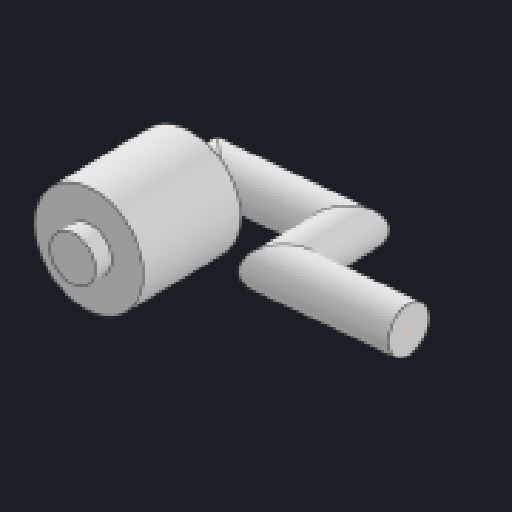
# Autodesk Inventor part: shoulder
Saved by Autodesk Inventor 2023 (Build 270158000, 158)
## iProperties
Created: 2024-02-21
Part Number: shoulder
Material: Generic
Document SubType Name: Modeling
Designer: valer
Density: 1 g/cm^3
Appearance: Default
Author: valer
Autodesk Inventor part; units mm, degrees
ref_plane "YZ Plane" through (0, 0, 0) normal (1, 0, 0) x (0, 1, 0)
ref_plane "XZ Plane" through (0, 0, 0) normal (0, 1, 0) x (-1, 0, 0)
ref_plane "XY Plane" through (0, 0, 0) normal (0, 0, 1) x (1, 0, 0)
sketch "LinkPath" plane through (0, 0, 0) normal (0, 0, 1) x (1, 0, 0)
  line L0 (0, 0) -> (0, 250)
  line L1 (0, 250) -> (350, 250)
  line L2 (350, 250) -> (350, 50)
  line L3 (350, 50) -> (700, 50)
  dimension "d26" = 250
  dimension "d27" = 350
  dimension "d28" = 200
  dimension "d29" = 350
  constraints: 8 end point, 3 perpendicular, 1 vertical
  measures "d26" distance of L0.start L0.end
  measures "d27" distance of L0.end L1.end
  measures "d28" distance of L1.end L2.end
  measures "d29" distance of L2.end L3.end
sketch "LinkProfile" plane through (0, 0, 0) normal (0, 1, 0) x (-1, 0, 0)
  circle A0 centre (0, 0) radius 62.5
  dimension "d30" = 125
  constraints: 1 centre point, 1 coincident
  measures "d30" diameter of A0
sweep "LinkFeature" add profiles "LinkProfile" path "LinkPath"
sketch "JointProfile" plane through (0, 0, 0) normal (0, -1, 0) x (1, 0, 0)
  circle A0 centre (0, 0) radius 150
  dimension "d33" = 300
  constraints: 1 centre point, 1 coincident
  measures "d33" diameter of A0
extrude "JointFeature" add sketch "JointProfile" along normal mid plane 300
sketch "JointAxis" plane through (0, -150, 0) normal (0, -1, 0) x (1, 0, 0)
  circle A0 centre (0, 0) radius 62.5
  dimension "d36" = 125
  constraints: 1 centre point, 1 coincident
  measures "d36" diameter of A0
extrude "JointAxisFeature" add sketch "JointAxis" along normal blind 50
sketch "Connection" plane through (700, 50, 0) normal (1, 0, 0) x (0, 0, -1)
  circle A0 centre (0, 0) radius 62.5 construction
  point P0 (0, -50)
  constraints: 1 coincident
body "Solid5"
